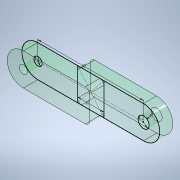
# Autodesk Inventor part: Biellette support-doigts
Saved by Autodesk Inventor 2022 (Build 260153000, 153)
## iProperties
Created: 2022-04-30
Part Number: Biellette support-doigts
Material: Générique
Document SubType Name: Modeling
Designer: victo
Density: 1 g/cm^3
Appearance: Transparent - Vert 1
Author: victo
Autodesk Inventor part; units mm, degrees
ref_plane "YZ Plane" through (0, 0, 0) normal (1, 0, 0) x (0, 1, 0)
ref_plane "XZ Plane" through (0, 0, 0) normal (0, 1, 0) x (-1, 0, 0)
ref_plane "XY Plane" through (0, 0, 0) normal (0, 0, 1) x (1, 0, 0)
sketch "Esquisse1" plane through (0, 0, 0) normal (0, 0, 1) x (1, 0, 0)
  line L0 (20, 0) -> (-20, 0) construction
  line L1 (20, -6.1) -> (-20, -6.1)
  line L2 (-20, 6.1) -> (20, 6.1)
  arc A0 (20, -6.1) -> (20, 6.1) centre (20, 0) ccw
  arc A1 (-20, 6.1) -> (-20, -6.1) centre (-20, 0) ccw
  circle A2 centre (-20, 0) radius 1.55
  circle A3 centre (20, 0) radius 2.1
  line L3 (-5, -6.1) -> (5, -6.1)
  line L4 (5, -6.1) -> (5, 6.1)
  line L5 (5, 6.1) -> (-5, 6.1)
  line L6 (-5, 6.1) -> (-5, -6.1)
  line L7 (-5, -6.1) -> (5, 6.1) construction
  line L8 (5, -6.1) -> (-5, 6.1) construction
  point P0 (0, 0)
  dimension "d0" = 40
  dimension "d1" = 3.1
  dimension "d5" = 4.2
  dimension "d6" = 4
  dimension "d12" = 10
  constraints: 20 end point, 4 centre point, 4 point on circle, 4 tangent, 3 midpoint, 3 parallel, 2 coincident, 2 horizontal, 1 perpendicular, 1 point on line
  measures "d0" distance of L0.end L0.start
  measures "d1" diameter of A2
  measures "d5" diameter of A3
  measures "d6" radial gap between concentric circles of A0 A3
  measures "d12" distance between parallel lines of L4 L6
extrude "Extrusion1" add sketch "Esquisse1" along normal blind 5.5 contours L1 L6 L2 L4 | L1 A1 L2 L6
extrude "Extrusion4" add sketch "Esquisse1" against normal blind 5 contours L1 L4 L2 A0 | L1 L6 L2 L4
fillet "Congé1" radius 1.5 4 edges at (-5, 6.1, -2.5) (-5, -6.1, -2.5) (5, -6.1, 2.75) (5, 6.1, 2.75)
